arms (Autodesk Fusion 360 design; units mm, degrees)
Autodesk Fusion 360 part; units mm, degrees
sketch "Sketch1" plane through (0, 0, 0) normal (0, 0, 1) x (1, 0, 0)
  line L0 (7.5, -25) -> (-7.5, -25)
  line L1 (-7.5, -25) -> (-7.5, 25)
  line L2 (7.5, 25) -> (7.5, -25)
  line L3 (7.5, -25) -> (-7.5, 25) construction
  line L4 (-7.5, -25) -> (7.5, 25) construction
  line L5 (-72.5, 25) -> (-72.5, 35)
  line L6 (-72.5, 35) -> (7.5, 35)
  line L7 (7.5, 35) -> (7.5, 25)
  line L8 (-72.5, 25) -> (-7.5, 25)
  circle A0 centre (-0.5, -19) radius 2.1
  circle A1 centre (-0.5, -9) radius 2.1
  dimension "d1" = 50
  dimension "d2" = 15
  dimension "d3" = 10
  dimension "d4" = 80
  dimension "d11" = 4.2
  dimension "d12" = 4.2
  dimension "d13" = 6
  dimension "d14" = 10
  dimension "d15" = 8
  dimension "d16" = 8
  dimension "d19" = 7
  constraint perpendicular L0 L1
  constraint parallel L1 L2
  constraint horizontal L0
  constraint coincident L3 origin
  constraint coincident L4 origin
  constraint vertical L5
  constraint horizontal L6
  constraint vertical L7
  constraint perpendicular L1 L8
  measures "d1" distance of L0.end L1.end
  measures "d2" distance of L1.end L2.start
  measures "d3" distance of L2.start L6.end
  measures "d4" distance of L5.end L6.end
  measures "d11" diameter of A0
  measures "d12" diameter of A1
  measures "d13" distance of L0 A0.centre
  measures "d14" vertical distance of A0.centre A1.centre
  measures "d15" distance of L2 A0.centre
  measures "d16" distance of L2 A1.centre
  measures "d19" distance of L1 A0.centre
extrude "Extrude1" add sketch "Sketch1" along normal blind 14
sketch "Sketch2" plane through (-7.5, 0, 0) normal (-1, 0, 0) x (0, -1, 0)
  line L0 (-25, 0) -> (25, 0)
  line L1 (25, 0) -> (25, 14)
  line L2 (25, 14) -> (-25, 14)
  line L3 (-25, 14) -> (-25, 0)
  line L4 (25, 12.1) -> (4.8, 12.1)
  line L5 (4.8, 12.1) -> (4.8, 1.9)
  line L6 (4.8, 1.9) -> (25, 1.9)
  line L7 (25, 1.9) -> (25, 12.1)
  line L8 (25, 14) -> (-25, 0) construction
  line L9 (-25, 14) -> (25, 0) construction
  line L10 (0, 7) -> (45, 7) construction
  dimension "d7" = 10.2
  dimension "d8" = 20.2
  constraint horizontal L4
  constraint vertical L5
  constraint horizontal L6
  constraint vertical L7
  constraint coincident L1 L4.start
  constraint coincident L1.end L2.start
  constraint coincident L0.start L3.end
  constraint coincident L2.end L3.start
  constraint coincident L0.end L1.start
  constraint midpoint L8 L10.start
  constraint perpendicular L1 L10
  constraint symmetric L4.start L6.end L10
  measures "d7" distance of L4.start L6.end
  measures "d8" distance of L4.start L4.end
extrude "Extrude2" cut sketch "Sketch2" against normal blind 13 contours L1 L4 L5 L6 L7
sketch "Sketch3" plane through (0, 35, 0) normal (0, 1, 0) x (-1, 0, 0)
  line L0 (-7.5, 0) -> (72.5, 0)
  line L1 (72.5, 0) -> (72.5, 14)
  line L2 (72.5, 14) -> (-7.5, 14)
  line L3 (-7.5, 14) -> (-7.5, 0)
fillet "Fillet1" radius 15 1 edges at (7.5, 35, 7)
fillet "Fillet1" radius 7.5 1 edges at (-7.5, 25, 7)
sketch "Sketch4" plane through (0, 35, 0) normal (0, 1, 0) x (-1, 0, 0)
  line L0 (59.5, 14) -> (59.5, 0) construction
  line L1 (7.5, 14) -> (7.5, 0)
  line L2 (7.5, 0) -> (72.5, 0)
  line L3 (72.5, 0) -> (72.5, 14)
  line L4 (72.5, 14) -> (7.5, 14)
  line L5 (72.5, 7) -> (1.5224, 7) construction
  circle A0 centre (59.5, 7) radius 6
  circle A1 centre (42.55, 7) radius 2.75
  circle A2 centre (76.45, 7) radius 2.75
  line L6 (39.8, 7) -> (39.8, 0) construction
  line L7 (79.2, 7) -> (79.2, 0) construction
  circle A3 centre (59.5, 7) radius 1.6
  circle A4 centre (59.5, 7) radius 5.25
  line L8 (42.1444, 9.7199) -> (58.7257, 12.1926)
  line L9 (42.1444, 4.2801) -> (58.7257, 1.8074)
  line L10 (76.8556, 4.2801) -> (60.2743, 1.8074)
  line L11 (76.8556, 9.7199) -> (60.2743, 12.1926)
  point P0 (-7.5, 14)
  dimension "d20" = 67
  dimension "d21" = 12
  dimension "d22" = 5.5
  dimension "d23" = 5.5
  dimension "d24" = 19.7
  dimension "d25" = 19.7
  dimension "d26" = 3.2
  dimension "d31" = 10.5
  constraint vertical L0
  constraint midpoint L3 L5.start
  constraint perpendicular L1 L5
  constraint midpoint L0 A0.centre
  constraint coincident L5 A1.centre
  constraint coincident L5 A2.centre
  constraint coincident A1 L6.start
  constraint coincident L5 L6.start
  constraint coincident L2 L6.end
  constraint tangent A1 L6
  constraint coincident A2 L7.start
  constraint coincident L5 L7.start
  constraint coincident L2 L7.end
  constraint tangent A2 L7
  constraint concentric A0 A3
  constraint coincident L5 A0.centre
  constraint coincident L0.end L2
  constraint concentric A3 A4
  constraint coincident A1 L8.start
  constraint coincident A4 L8.end
  constraint tangent A4 L8
  constraint coincident A1 L9.start
  constraint coincident A4 L9.end
  constraint tangent A4 L9
  constraint coincident A2 L10.start
  constraint coincident A4 L10.end
  constraint tangent A4 L10
  constraint coincident A2 L11.start
  constraint coincident A4 L11.end
  constraint tangent A4 L11
  constraint tangent A2 L11
  constraint tangent A2 L10
  constraint tangent A1 L8
  constraint tangent A1 L9
  measures "d20" distance of L0.start P0
  measures "d21" diameter of A0
  measures "d22" diameter of A1
  measures "d23" diameter of A2
  measures "d24" distance of L0.end L6.end
  measures "d25" distance of L0.end L7.end
  measures "d26" diameter of A3
  measures "d31" diameter of A4
extrude "Extrude3" cut sketch "Sketch4" against normal blind 5 contours L3 A2 L10 L11 | L3 A0 L10 L11 | A2 | A0 A4 L8 L11 | A0 A4 L10 L11 | A0 A4 L9 L10 | A0 A4 L8 L9 | A0 A1 L8 L9 | A4 | A1
extrude "Extrude4" cut 1 faces at (-60.4127, 35, 7.0214) along direction (0, -1, 0) through all
ref_plane "WorkPlane1" through (-33.5, 0, 7) normal (1, 0, 0) x (0, 1, 0)
split "Split1" [suppressed]
